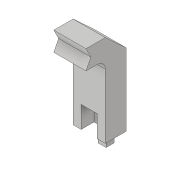
# Autodesk Inventor part: 3point finger
Saved by Autodesk Inventor 2017 (Build 210142000, 142)
## iProperties
Created: 2017-12-10
Part Number: 3point finger
Material: Generic
Document SubType Name: Modeling
Designer: Jeyy
Density: 1 g/cm^3
Appearance: Default
Author: Jeyy
Autodesk Inventor part; units mm, degrees
ref_plane "YZ Plane" through (0, 0, 0) normal (1, 0, 0) x (0, 1, 0)
ref_plane "XZ Plane" through (0, 0, 0) normal (0, 1, 0) x (-1, 0, 0)
ref_plane "XY Plane" through (0, 0, 0) normal (0, 0, 1) x (1, 0, 0)
sketch "Sketch2" plane through (0, 0, 0) normal (1, 0, 0) x (0, 1, 0)
  line L0 (0, 0) -> (15, 0)
  line L1 (15, 0) -> (15, -10)
  line L2 (15, -10) -> (0, -10)
  line L3 (0, -10) -> (0, 0)
  dimension "d4" = 15
  dimension "d5" = 10
  constraints: 8 end point, 2 parallel, 1 horizontal, 1 perpendicular
  measures "d4" distance of L1.end L2.end
  measures "d5" distance of L0.end L1.end
extrude "Extrusion2" add sketch "Sketch2" along normal blind 12
sketch "Sketch3" plane through (0, 0, 0) normal (0, 0, 1) x (1, 0, 0)
  line L0 (0, 0) -> (1, 0)
  line L1 (0, 0) -> (12, 0) projected
  line L2 (1, 0) -> (1, 13.5)
  line L3 (1, 13.5) -> (11, 13.5)
  line L4 (11, 13.5) -> (11, 0)
  line L5 (11, 0) -> (1, 0)
  dimension "d8" = 1
  dimension "d9" = 13.5
  dimension "d10" = 10
  constraints: 10 end point, 3 perpendicular, 2 point on line, 1 vertical
  measures "d8" distance of L0.start L0.end
  measures "d9" distance of L0.end L2.end
  measures "d10" distance of L2.end L3.end
extrude "Extrusion3" cut sketch "Sketch3" against normal blind 8
sketch "Sketch4" plane through (0, 0, -10) normal (0, 0, -1) x (-1, 0, 0)
  line L0 (0, 15) -> (-12, 15) projected
  line L1 (0, 0) -> (-12, 0) projected
  line L2 (-12, 15) -> (0, 15)
  line L3 (0, 15) -> (0, 0)
  line L4 (0, 0) -> (-12, 0)
  line L5 (-12, 0) -> (-12, 15)
  constraints: 8 end point, 2 parallel, 1 horizontal, 1 perpendicular
extrude "Extrusion4" add sketch "Sketch4" along normal blind 2
sketch "Sketch5" plane through (0, 0, -8) normal (0, 0, 1) x (1, 0, 0)
  line L0 (1, 13.5) -> (11, 13.5) projected
  line L1 (6, 13.5) -> (6, 10)
  line L2 (6, 10) -> (6, 3.5)
  circle A0 centre (6, 10) radius 1.2295
  circle A1 centre (6, 3.5) radius 1.2295
  point P0 (0, 0)
  dimension "d15" = 3.5
  dimension "d16" = 6.5
  dimension "d17" = 2.459
  dimension "d18" = 2.459
  constraints: 4 end point, 2 centre point, 2 coincident, 1 midpoint, 1 point on line, 1 vertical
  measures "d15" distance of L1.start L1.end
  measures "d16" distance of L1.end L2.end
  measures "d17" diameter of A0
  measures "d18" diameter of A1
extrude "Extrusion5" cut sketch "Sketch5" against normal blind 4
sketch "Sketch6" plane through (0, 0, -8) normal (0, 0, 1) x (1, 0, 0)
  circle A0 centre (6, 10) radius 1.2295 projected
  circle A1 centre (6, 10) radius 2.7
  circle A2 centre (6, 3.5) radius 1.2295 projected
  circle A3 centre (6, 3.5) radius 2.7
  point P0 (0, 0)
  dimension "d21" = 5.4
  dimension "d22" = 5.4
  constraints: 2 centre point, 2 coincident
  measures "d21" diameter of A1
  measures "d22" diameter of A3
extrude "Extrusion6" cut sketch "Sketch6" against normal blind 1.1
sketch "Sketch15" plane through (12, 0, 0) normal (1, 0, 0) x (0, 0, -1)
  line L0 (0, 15) -> (12, 15) projected
  line L1 (12, 15) -> (12, 0) projected
  line L2 (0, 15) -> (12, 15)
  line L3 (12, 15) -> (12, 0)
  line L4 (12, 0) -> (0, 0)
  line L5 (0, 0) -> (0, 15)
  constraints: 8 end point, 2 parallel, 1 horizontal, 1 perpendicular
extrude "Extrusion14" add sketch "Sketch15" along normal blind 4
ref_plane "Work Plane1" through (6, 0, 0) normal (1, 0, 0) x (0, 0, -1)
mirror "Mirror1" about plane through (6, 0, 0) normal (1, 0, 0) of "Extrusion14"
sketch "Sketch16" plane through (1, 0, -8) normal (0, -1, 0) x (1, 0, 0)
  line L0 (10, 0) -> (0, 0) projected
  line L1 (5, 0) -> (7.5, 0)
  line L2 (7.5, 0) -> (7.5, -4)
  line L3 (-5, -4) -> (15, -4) projected
  line L4 (7.5, -4) -> (2.5, -4)
  line L5 (2.5, -4) -> (2.5, 0)
  line L6 (2.5, 0) -> (5, 0)
  point P0 (-1, 8)
  dimension "d61" = 2.5
  dimension "d62" = 4
  dimension "d63" = 5
  dimension "d64" = 4
  constraints: 10 end point, 4 point on line, 1 midpoint, 1 perpendicular
  measures "d61" distance of L1.start L1.end
  measures "d62" distance of L1.end L2.end
  measures "d63" distance of L2.end L4.end
  measures "d64" distance of L4.end L5.end
extrude "Extrusion15" add sketch "Sketch16" along normal blind 10
sketch "Sketch18" plane through (0, 0, -12) normal (0, 0, -1) x (-1, 0, 0)
  line L0 (-16, 15) -> (4, 15) projected
  line L1 (4, 0) -> (-3.5, 0) projected
  line L2 (-16, 15) -> (4, 15)
  line L3 (4, 15) -> (4, 0)
  line L4 (4, 0) -> (-16, 0)
  line L5 (-16, 0) -> (-16, 15)
  line L6 (-8.5, -10) -> (-3.5, -10) projected
  line L7 (-3.5, 0) -> (-8.5, 0)
  line L8 (-8.5, 0) -> (-8.5, -10)
  line L9 (-8.5, -10) -> (-3.5, -10)
  line L10 (-3.5, -10) -> (-3.5, 0)
  circle A0 centre (-6, 3.5) radius 1.2295 projected
  circle A1 centre (-6, 3.5) radius 1.2295
  circle A2 centre (-6, 10) radius 1.2295 projected
  circle A3 centre (-6, 10) radius 1.2295
  point P0 (0, 0)
  constraints: 16 end point, 4 parallel, 2 centre point, 2 coincident, 2 horizontal, 2 perpendicular
extrude "Extrusion16" add sketch "Sketch18" along normal blind 1
sketch "Sketch19" plane through (16, 0, 0) normal (1, 0, 0) x (0, 0, -1)
  line L0 (0, 15) -> (13, 15) projected
  line L1 (0, 15) -> (0, 40)
  line L2 (-5, 45) -> (-12, 45)
  line L3 (13, 45) -> (13, 15)
  line L4 (0, 57) -> (-12, 57)
  line L5 (0, 57) -> (13, 45)
  line L6 (-9, 51) -> (-12, 57)
  line L7 (-9, 51) -> (-12, 45)
  arc A0 (0, 40) -> (-5, 45) centre (-5, 40) ccw
  point P0 (0, 0)
  point P1 (0, 45)
  dimension "d69" = 30
  dimension "d75" = 5
  constraints: 14 end point, 2 point on circle, 2 point on line, 2 tangent, 1 centre point, 1 horizontal, 1 perpendicular, 1 vertical
  measures "d69" distance of L0.start point (0, 45)
  measures "d75" radius of A0
extrude "Extrusion17" add sketch "Sketch19" against normal blind 20
thread "Thread1" size "M3x0.5" class "6H" standard "ANSI Metric M Profile" full length
thread "Thread2" size "M3x0.5" class "6H" standard "ANSI Metric M Profile" full length
body "Solid2"
